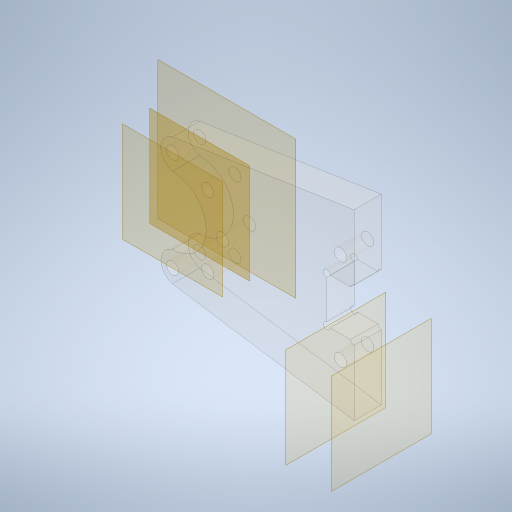
# Autodesk Inventor part: feet_holder1
Saved by Autodesk Inventor 2024 (Build 280153000, 153)
## iProperties
Created: 2024-09-03
Part Number: feet_holder1
Material: PMMA 플라스틱
Document SubType Name: Modeling
Designer: jmha0
Density: 1.188 g/cm^3
Appearance: 폴리카보네이트 - 선명
Author: jmha0
Autodesk Inventor part; units mm, degrees
ref_plane "YZ Plane" through (0, 0, 0) normal (1, 0, 0) x (0, 1, 0)
ref_plane "XZ Plane" through (0, 0, 0) normal (0, 1, 0) x (-1, 0, 0)
ref_plane "XY Plane" through (0, 0, 0) normal (0, 0, 1) x (1, 0, 0)
ref_plane "작업 평면1" through (0, 0, 0) normal (0, 0, 1) x (1, 0, 0)
ref_plane "작업 평면3" through (0, 0, 6) normal (0, 0, 1) x (1, 0, 0)
ref_plane "작업 평면4" through (40, -20.1, 6) normal (1, 0, 0) x (0, 0, -1)
ref_plane "작업 평면2" through (0, 0, 6) normal (0, 0, 1) x (1, 0, 0)
ref_plane "작업 평면6" through (30, -20.1, 6) normal (1, 0, 0) x (0, 0, -1)
ref_plane "작업 평면5" through (0, 0, 12) normal (0, 0, 1) x (1, 0, 0)
sketch "스케치6" plane through (0, 0, 12) normal (0, 0, 1) x (1, 0, 0)
  arc A0 (0, -7.45) -> (0, 7.45) centre (0, 0) ccw
  arc A1 (0, -7.45) -> (0, -14) centre (0.8514, -10.725) ccw
  line L0 (40, -20.1) -> (0, -14)
  line L1 (40, 20.1) -> (40, -20.1)
  line L2 (0, 14) -> (40, 20.1)
  arc A2 (0, 14) -> (0, 7.45) centre (0.8364, 10.725) ccw
  circle A3 centre (0, -11) radius 1.35
  circle A4 centre (7.7782, -7.7782) radius 1.35
  circle A5 centre (11, 0) radius 1.35
  circle A6 centre (7.7782, 7.7782) radius 1.35
  circle A7 centre (0, 11) radius 1.35
  constraints: 8 centre point, 6 end point, 6 point on circle
extrude "돌출6" add sketch "스케치6" against normal blind 6
sketch "스케치9" plane through (0, 0, 12) normal (0, 0, 1) x (1, 0, 0)
  arc A0 (0, -7.45) -> (0, 7.45) centre (0, 0) ccw projected
  arc A1 (0, -7.45) -> (0, -14) centre (0.8514, -10.725) ccw projected
  line L0 (0, -14) -> (40, -20.1) projected
  line L1 (40, -20.1) -> (40, 20.1) projected
  line L2 (40, 20.1) -> (0, 14) projected
  arc A2 (0, 14) -> (0, 7.45) centre (0.8364, 10.725) ccw projected
  circle A3 centre (11, 0) radius 1.35 projected
  circle A4 centre (0, 11) radius 1.35 projected
  circle A5 centre (7.7782, 7.7782) radius 1.35 projected
  circle A6 centre (7.7782, -7.7782) radius 1.35 projected
  circle A7 centre (0, -11) radius 1.35 projected
  line L3 (40, 20.1) -> (40, -20.1)
  line L4 (40, -20.1) -> (34, -20.1)
  line L5 (34, -20.1) -> (34, 20.1)
  line L6 (34, 20.1) -> (40, 20.1)
  line L7 (40, 20.1) -> (40, 10.05)
  line L8 (40, 10.05) -> (40, -10.05)
  circle A8 centre (37, 10.05) radius 1.35
  circle A9 centre (37, -10.05) radius 1.35
  dimension "d41" = 6
  dimension "d42" = 10.05
  dimension "d43" = 20.1
  dimension "d44" = 2.7
  dimension "d45" = 2.7
  constraints: 12 end point, 3 equal length, 2 centre point, 2 point on line, 1 perpendicular
  measures "d41" distance of L0.end L4.end
  measures "d42" distance of L1.end L7.end
  measures "d43" distance of L7.end L8.end
  measures "d44" diameter of A8
  measures "d45" diameter of A9
extrude "돌출8" cut sketch "스케치9" against normal blind 6 contours A8 | A9
sketch "스케치10" plane through (0, 0, 12) normal (0, 0, 1) x (1, 0, 0)
  circle A0 centre (37, -10.05) radius 1.35 projected
  circle A1 centre (37, 10.05) radius 1.35 projected
  arc A2 (0, -7.45) -> (0, 7.45) centre (0, 0) ccw projected
  arc A3 (0, -7.45) -> (0, -14) centre (0.8514, -10.725) ccw projected
  line L0 (0, -14) -> (40, -20.1) projected
  line L1 (40, -20.1) -> (40, 20.1) projected
  line L2 (40, 20.1) -> (0, 14) projected
  arc A4 (0, 14) -> (0, 7.45) centre (0.8364, 10.725) ccw projected
  circle A5 centre (11, 0) radius 1.35 projected
  circle A6 centre (0, 11) radius 1.35 projected
  circle A7 centre (7.7782, 7.7782) radius 1.35 projected
  circle A8 centre (7.7782, -7.7782) radius 1.35 projected
  circle A9 centre (0, -11) radius 1.35 projected
  line L3 (34, -5) -> (40, -5)
  line L4 (40, -5) -> (40, 5)
  line L5 (40, 5) -> (34, 5)
  line L6 (34, 5) -> (34, -5)
  line L7 (34, -5) -> (40, 5) construction
  line L8 (40, -5) -> (34, 5) construction
  circle A10 centre (40, 5) radius 0.75
  circle A11 centre (34, 5) radius 0.75
  circle A12 centre (34, -5) radius 0.75
  circle A13 centre (40, -5) radius 0.75
  point P0 (37, 0)
  point P1 (39.25, -5)
  point P2 (40, -5.75)
  point P3 (34, -4.25)
  point P4 (34.75, -5)
  point P5 (34.75, 5)
  point P6 (34, 4.25)
  point P7 (40, 5.75)
  point P8 (39.25, 5)
  dimension "d48" = 10
  dimension "d51" = 1.5
  dimension "d52" = 1.5
  dimension "d53" = 1.5
  dimension "d54" = 1.5
  constraints: 12 end point, 4 centre point, 4 coincident, 2 midpoint, 2 parallel, 1 horizontal, 1 perpendicular, 1 point on line
  measures "d48" distance of L4.end L3.end
  measures "d51" diameter of A10
  measures "d52" diameter of A11
  measures "d53" diameter of A12
  measures "d54" diameter of A13
extrude "돌출9" cut sketch "스케치10" against normal blind 10 contours A13 L3 L1 | L1 L5 A10 | L3 A13 L1 | L3 A12 L6 A11 L5 A10 L1 A13 | L1 A10 L5 | A12 L6 L3 | L3 L6 A12 | A11 L6 L5 | L5 L6 A11
